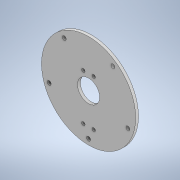
# Autodesk Inventor part: Base2
Saved by Autodesk Inventor 2022 (Build 260153000, 153)
## iProperties
Created: 2021-09-09
Part Number: Base2
Material: Generic
Document SubType Name: Modeling
Designer: Administrador
Density: 1 g/cm^3
Appearance: Default
Author: Administrador
Autodesk Inventor part; units mm, degrees
ref_plane "YZ Plane" through (0, 0, 0) normal (1, 0, 0) x (0, 1, 0)
ref_plane "XZ Plane" through (0, 0, 0) normal (0, 1, 0) x (-1, 0, 0)
ref_plane "XY Plane" through (0, 0, 0) normal (0, 0, 1) x (1, 0, 0)
sketch "Sketch1" plane through (0, 0, 0) normal (0, 0, 1) x (1, 0, 0)
  circle A0 centre (0, 0) radius 50
  circle A1 centre (0, 0) radius 11.75
  circle A2 centre (0, -44) radius 2.1
  circle A3 centre (-41.8465, -13.5967) radius 2.1
  circle A4 centre (-25.8626, 35.5967) radius 2.1
  circle A5 centre (25.8626, 35.5967) radius 2.1
  circle A6 centre (41.8465, -13.5967) radius 2.1
  line L0 (25.8626, 35.5967) -> (30.8626, 35.5967) construction
  line L1 (25.8626, 35.5967) -> (31.8626, 35.5967) construction
  circle A7 centre (-5.5, 16) radius 1.8
  circle A8 centre (5.5, 16) radius 1.8
  circle A9 centre (5.5, -33) radius 1.8
  circle A10 centre (-5.5, -33) radius 1.8
  line L2 (0, 50) -> (-5.5, 50) construction
  dimension "d0" = 100
  dimension "d3" = 23.5
  dimension "d7" = 4.2
  dimension "d8" = 4.2
  dimension "d9" = 4.2
  dimension "d10" = 4.2
  dimension "d11" = 4.2
  dimension "d18" = 3.6
  dimension "d21" = 34
  dimension "d22" = 11
  dimension "d23" = 49
  dimension "d24" = 49
  dimension "d25" = 11
  constraints: 10 centre point, 6 end point, 4 horizontal, 2 coincident, 1 vertical alignment, 2 other
  measures "d3" diameter of A1
  measures "d7" diameter of A2
  measures "d8" diameter of A3
  measures "d9" diameter of A4
  measures "d10" diameter of A5
  measures "d11" diameter of A6
  measures "d18" diameter of A7
  measures "d21" distance from line of A7.centre L2
  measures "d22" distance of A8.centre A7.centre
  measures "d23" distance of A9.centre A8.centre
  measures "d24" distance of A7.centre A10.centre
  measures "d25" distance of A9.centre A10.centre
extrude "Extrusion1" add sketch "Sketch1" along normal blind 3
body "Solid1"
